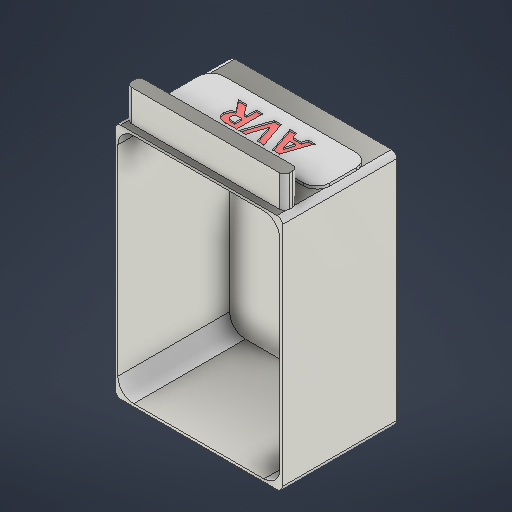
# Autodesk Inventor part: shelf
Saved by Autodesk Inventor 2027 (Build 310192060, 192F)
## iProperties
Created: 2026-06-08
Part Number: shelf
Material: Ogólny
Document SubType Name: Modeling
Designer: User
Density: 1 g/cm^3
Appearance: Domyślna
Author: User
Autodesk Inventor part; units mm, degrees
ref_plane "YZ Plane" through (0, 0, 0) normal (1, 0, 0) x (0, 1, 0)
ref_plane "XZ Plane" through (0, 0, 0) normal (0, 1, 0) x (-1, 0, 0)
ref_plane "XY Plane" through (0, 0, 0) normal (0, 0, 1) x (1, 0, 0)
sketch "Szkic1" plane through (0, 0, 0) normal (0, 1, 0) x (-1, 0, 0)
  line L0 (-31.7, -21.7) -> (31.7, -21.7)
  line L1 (31.7, -21.7) -> (31.7, 21.7)
  line L2 (31.7, 21.7) -> (-31.7, 21.7)
  line L3 (-31.7, 21.7) -> (-31.7, -21.7)
  line L4 (-31.7, -21.7) -> (31.7, 21.7) construction
  line L5 (31.7, -21.7) -> (-31.7, 21.7) construction
  point P0 (0, 0)
  dimension "d0" = 63.4
  dimension "d1" = 43.4
  constraints: 12 end point, 2 midpoint, 2 parallel, 1 horizontal, 1 perpendicular
  measures "d0" distance of L2.end L1.end
  measures "d1" distance of L1.end L0.end
extrude "Wyciągnięcie proste1" add sketch "Szkic1" along normal blind 90
shell "Skorupa1" thickness 1 removed faces 1 at (-10.5667, 30, 21.7)
sketch "Szkic2" plane through (0, 90, 0) normal (0, 1, 0) x (1, 0, 0)
  line L0 (-31.7, -21.7) -> (31.7, -21.7) projected
  line L1 (0, -21.7) -> (0, -16.7)
  line L2 (30, -19.2) -> (-30, -19.2)
  line L3 (-30, -19.2) -> (-30, -14.2)
  line L4 (-30, -14.2) -> (30, -14.2)
  line L5 (30, -14.2) -> (30, -19.2)
  line L6 (30, -19.2) -> (-30, -14.2) construction
  line L7 (-30, -19.2) -> (30, -14.2) construction
  point P0 (0, 0)
  dimension "d5" = 5
  dimension "d6" = 60
  dimension "d7" = 5
  constraints: 14 end point, 3 midpoint, 2 parallel, 1 horizontal, 1 perpendicular, 1 vertical
  measures "d5" distance of L1.start L1.end
  measures "d6" distance of L2.start L2.end
  measures "d7" distance of L2.end L3.end
extrude "Wyciągnięcie proste2" add sketch "Szkic2" along normal blind 12
sketch "Szkic3" plane through (0, 90, 0) normal (0, 1, 0) x (1, 0, 0)
  line L0 (0, 0) -> (0, 3)
  line L1 (30, 13) -> (-30, 13)
  line L2 (-30, 13) -> (-30, -7)
  line L3 (-30, -7) -> (30, -7)
  line L4 (30, -7) -> (30, 13)
  line L5 (30, 13) -> (-30, -7) construction
  line L6 (-30, 13) -> (30, -7) construction
  dimension "d10" = 3
  dimension "d11" = 60
  dimension "d12" = 20
  constraints: 14 end point, 2 midpoint, 2 parallel, 1 horizontal, 1 perpendicular, 1 vertical
  measures "d10" distance of L0.start L0.end
  measures "d11" distance of L3.end L2.end
  measures "d12" distance of L2.end L1.end
extrude "Wyciągnięcie proste3" add sketch "Szkic3" along normal blind 1
sketch "Szkic4" plane through (0, 91, 0) normal (0, 1, 0) x (1, 0, 0)
  line L0 (30, -7) -> (-30, -7) construction
  line L1 (-30, -7) -> (-30, 13) construction
  line L2 (-30, 13) -> (30, 13) construction
  line L3 (30, 13) -> (30, -7) construction
  line L4 (-30, -7) -> (30, -7) projected
  line L5 (-30, 13) -> (-30, -7) projected
  line L6 (30, -7) -> (-30, -7)
  line L7 (-30, -7) -> (-30, 13)
  line L8 (-30, 13) -> (30, 13)
  line L9 (30, 13) -> (30, -7)
  line L10 (14.3801, 8) -> (11.0008, -2)
  line L11 (11.0008, -2) -> (8.2618, -2)
  line L12 (8.2618, -2) -> (4.8825, 8)
  line L13 (4.8825, 8) -> (7.4676, 8)
  line L14 (7.4676, 8) -> (8.0916, 5.9579)
  line L15 (8.0916, 5.9579) -> (11.2358, 5.9579)
  line L16 (11.2358, 5.9579) -> (11.8679, 8)
  line L17 (11.8679, 8) -> (14.3801, 8)
  line L18 (8.6426, 4.1426) -> (9.6637, 0.8363)
  line L19 (9.6637, 0.8363) -> (10.6929, 4.1426)
  line L20 (10.6929, 4.1426) -> (8.6426, 4.1426)
  line L21 (-4.4611, -2) -> (-1.0251, 8)
  line L22 (-1.0251, 8) -> (1.5924, 8)
  line L23 (1.5924, 8) -> (5.0284, -2)
  line L24 (5.0284, -2) -> (2.4271, -2)
  line L25 (2.4271, -2) -> (0.2472, 4.7828)
  line L26 (0.2472, 4.7828) -> (-1.9246, -2)
  line L27 (-1.9246, -2) -> (-4.4611, -2)
  line L28 (-14.6313, 8) -> (-11.5762, 8)
  line L29 (-11.5762, 8) -> (-8.7966, 4.329)
  line L30 (-8.7966, 4.329) -> (-7.889, 4.329)
  line L31 (-7.889, 4.329) -> (-7.889, 8)
  line L32 (-7.889, 8) -> (-5.393, 8)
  line L33 (-5.393, 8) -> (-5.393, -2)
  line L34 (-5.393, -2) -> (-9.4125, -2)
  spline S0 degree 2 poles (-9.4125, -2) (-10.2472, -2) (-11.4789, -1.7893) (-12.0057, -1.4652) knots 0 0 0 1 2 2 2
  spline S1 degree 2 poles (-12.0057, -1.4652) (-12.5405, -1.1248) (-13.1726, -0.0632) (-13.1726, 0.7472) knots 0 0 0 1 2 2 2
  spline S2 degree 2 poles (-13.1726, 0.7472) (-13.1726, 1.8898) (-12.1353, 3.3241) (-11.2682, 3.7455) knots 0 0 0 1 2 2 2
  line L35 (-11.2682, 3.7455) -> (-14.6313, 8)
  spline S3 degree 2 poles (-10.5956, 1.0632) (-10.5956, 0.6823) (-10.3039, 0.1394) (-9.9716, -0.0065) knots 0 0 0 1 2 2 2
  spline S4 degree 2 poles (-9.9716, -0.0065) (-9.7366, -0.1037) (-9.1613, -0.1605) (-8.7318, -0.1605) knots 0 0 0 1 2 2 2
  line L36 (-8.7318, -0.1605) -> (-7.889, -0.1605)
  line L37 (-7.889, -0.1605) -> (-7.889, 2.53)
  line L38 (-7.889, 2.53) -> (-8.6102, 2.53)
  spline S5 degree 2 poles (-8.6102, 2.53) (-9.1288, 2.53) (-9.8663, 2.4003) (-10.1175, 2.1977) knots 0 0 0 1 2 2 2
  spline S6 degree 2 poles (-10.1175, 2.1977) (-10.3606, 2.0032) (-10.5956, 1.4846) (-10.5956, 1.0632) knots 0 0 0 1 2 2 2
  point P0 (0, 0)
  dimension "d0" = 63.4
  dimension "d1" = 43.4
  constraints: 8 end point, 2 coincident, 2 parallel, 1 horizontal, 1 perpendicular, 2 other
extrude "Wyciągnięcie proste4" cut sketch "Szkic4" against normal blind 0.6 contours L10 L11 L12 L13 L14 L15 L16 L17 | L21 L22 L23 L24 L25 L26 L27 | L28 L29 L30 L31 L32 L33 L34 S0 S1 S2 L35
fillet "Zaokrąglenie1" radius 5 4 edges at (-30, 90.5, 7) (-30, 90.5, -13) (30, 90.5, 7) (30, 90.5, -13)
fillet "Zaokrąglenie2" radius 6 4 edges at (30.7, 1, 0.5) (-30.7, 1, 0.5) (30.7, 89, 0.5) (-30.7, 89, 0.5)
fillet "Zaokrąglenie3" radius 2 4 edges at (31.7, 90, 0) (-31.7, 90, 0) (-31.7, 0, 0) (31.7, 0, 0)
fillet "Zaokrąglenie4" radius 2 4 edges at (-30, 95.9887, 14.2) (-30, 95.9887, 19.2) (30, 95.9887, 14.2) (30, 95.9887, 19.2)
